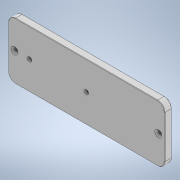
# Autodesk Inventor part: Base Plate
Saved by Autodesk Inventor 2020 (Build 240168000, 168)
## iProperties
Created: 2020-01-31
Part Number: Base Plate
Material: Generic
Document SubType Name: Modeling
Designer: cks4a449
Density: 1 g/cm^3
Appearance: Default
Author: cks4a449
Autodesk Inventor part; units mm, degrees
ref_plane "YZ Plane" through (0, 0, 0) normal (1, 0, 0) x (0, 1, 0)
ref_plane "XZ Plane" through (0, 0, 0) normal (0, 1, 0) x (-1, 0, 0)
ref_plane "XY Plane" through (0, 0, 0) normal (0, 0, 1) x (1, 0, 0)
sketch "Sketch1" plane through (0, 0, 0) normal (0, 0, 1) x (1, 0, 0)
  line L0 (12.7, 0) -> (266.7, 0)
  line L1 (279.4, 12.7) -> (279.4, 88.9)
  line L2 (266.7, 101.6) -> (12.7, 101.6)
  line L3 (0, 88.9) -> (0, 12.7)
  arc A0 (12.7, 101.6) -> (0, 88.9) centre (12.7, 88.9) ccw
  arc A1 (0, 12.7) -> (12.7, 0) centre (12.7, 12.7) ccw
  arc A2 (266.7, 0) -> (279.4, 12.7) centre (266.7, 12.7) ccw
  arc A3 (279.4, 88.9) -> (266.7, 101.6) centre (266.7, 88.9) ccw
  point P0 (0, 0)
  point P1 (279.4, 101.6)
  point P2 (279.4, 0)
  point P3 (0, 101.6)
  dimension "d0" = 279.4
  dimension "d1" = 101.6
  dimension "d2" = 12.7
  constraints: 8 end point, 8 point on circle, 8 point on line, 8 tangent, 4 centre point, 3 equal radius, 2 parallel, 1 horizontal, 1 perpendicular
  measures "d0" distance of point (0, 101.6) point (279.4, 101.6)
  measures "d1" distance of point (279.4, 101.6) point (279.4, 0)
  measures "d2" radius of A0
extrude "Extrusion1" add sketch "Sketch1" along normal blind 12.7
chamfer "Chamfer1" distance 0.7937 angle 45 16 edges at (139.7, 101.6, 12.7) (3.7197, 97.8803, 12.7) (0, 50.8, 12.7) (3.7197, 3.7197, 12.7) (139.7, 0, 12.7) (275.6803, 3.7197, 12.7) (279.4, 50.8, 12.7) (275.6803, 97.8803, 12.7) (139.7, 101.6, 0) (3.7197, 97.8803, 0) (0, 50.8, 0) (3.7197, 3.7197, 0) (139.7, 0, 0) (275.6803, 3.7197, 0) (279.4, 50.8, 0) (275.6803, 97.8803, 0)
sketch "Sketch2" plane through (0, 0, 12.7) normal (0, 0, 1) x (1, 0, 0)
  line L0 (0.7937, 12.7) -> (0.7938, 88.9) projected
  line L1 (0, 88.9) -> (0, 12.7) projected
  line L2 (266.7, 101.6) -> (12.7, 101.6) projected
  line L3 (279.4, 12.7) -> (279.4, 88.9) projected
  point P0 (0, 0)
  point P1 (11.1125, 50.8)
  point P2 (38.1, 50.8)
  point P3 (139.7, 50.8)
  point P4 (268.2875, 50.8)
  dimension "d9" = 11.1125
  dimension "d10" = 50.8
  dimension "d11" = 50.8
  dimension "d12" = 50.8
  dimension "d13" = 50.8
  dimension "d14" = 11.1125
  dimension "d15" = 139.7
  dimension "d16" = 38.1
  measures "d9" distance from line of point (11.113, 50.8) L1
  measures "d10" distance from line of L2 point (11.113, 50.8)
  measures "d11" distance from line of L2 point (38.1, 50.8)
  measures "d12" distance from line of L2 point (139.7, 50.8)
  measures "d13" distance from line of L2 point (268.288, 50.8)
  measures "d14" distance from line of L3 point (268.288, 50.8)
  measures "d15" distance from line of L1 point (139.7, 50.8)
  measures "d16" distance from line of L1 point (38.1, 50.8)
hole "Hole1" at (11.1125, 50.8, 12.7) at (268.2875, 50.8, 12.7) direction (0, 0, -1) diameter 6.35 end through all countersink diameter 12.7 countersink angle 82
hole "Hole2" at (38.1, 50.8, 12.7) at (139.7, 50.8, 12.7) direction (0, 0, -1) diameter 7.9375 end through all
sketch "Sketch3" plane through (0, 0, 0) normal (0, 0, -1) x (-1, 0, 0)
  arc A0 (-12.7, 0.7937) -> (-0.7938, 12.7) centre (-12.7, 12.7) ccw projected
  arc A1 (-0.7938, 88.9) -> (-12.7, 100.8062) centre (-12.7, 88.9) ccw projected
  arc A2 (-266.7, 100.8062) -> (-278.6063, 88.9) centre (-266.7, 88.9) ccw projected
  arc A3 (-278.6063, 12.7) -> (-266.7, 0.7938) centre (-266.7, 12.7) ccw projected
  point P0 (0, 0)
  constraints: 4 coincident
hole "Hole3" at (12.7, 12.7, 0) at (12.7, 88.9, 0) at (266.7, 88.9, 0) at (266.7, 12.7, 0) direction (0, 0, 1) diameter 3.302 depth 7.3025 thread size "8-32 UNC" class "2B" standard "ANSI Unified Screw Threads"
body "Solid1"
